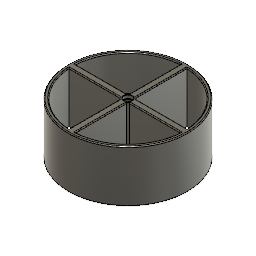
ExtrudedWheel v2 (Autodesk Fusion 360 design; units mm, degrees)
Autodesk Fusion 360 part; units mm, degrees
sketch "Sketch6" plane through (0, 0, 0) normal (0, 1, 0) x (1, 0, 0)
  circle A0 centre (0, 0) radius 73.5
  circle A1 centre (0, 0) radius 7
  circle A2 centre (0, 0) radius 71
  line L0 (4, 70.9044) -> (-4, 70.9044)
  line L1 (-4, 70.9044) -> (-4, -70.9044)
  line L2 (-4, -70.9044) -> (4, -70.9044)
  line L3 (4, -70.9044) -> (4, 70.9044)
  line L4 (4, 70.9044) -> (-4, -70.9044) construction
  line L5 (-4, 70.9044) -> (4, -70.9044) construction
  line L6 (72.9182, 4) -> (-72.9182, 4)
  line L7 (-72.9182, 4) -> (-72.9182, -4)
  line L8 (-72.9182, -4) -> (72.9182, -4)
  line L9 (72.9182, -4) -> (72.9182, 4)
  line L10 (72.9182, 4) -> (-72.9182, -4) construction
  line L11 (-72.9182, 4) -> (72.9182, -4) construction
  circle A3 centre (0, 0) radius 69
  dimension "d17" = 147
  dimension "d18" = 14
  dimension "d19" = 142
  dimension "d20" = 8
  dimension "d21" = 8
  dimension "d22" = 138
  measures "d17" diameter of A0
  measures "d18" diameter of A1
  measures "d19" diameter of A2
  measures "d22" diameter of A3
extrude "Extrude3" add sketch "Sketch6" along normal blind 64 contours A0 | A1 L3 L6 L8 | A1 L6 L8 A3 | A1 L3 L6 | A1 L3 L8 | A1 L1 L3 L6 | A1 L1 L3 A3 | A2 L3 L6 A3 | A2 L6 L8 A3 | L1 L3 L6 L8 | A1 L1 L3 A3 | A1 L1 L3 L8 | A2 L3 L8 A3 | A1 L1 L6 | A2 L0 L1 L3 A3 | A2 L6 L8 L9 | A1 L1 L6 L8 | A1 L1 L8 | A2 L1 L2 L3 A3 | A1 L6 L8 A3 | A2 L1 L6 A3 | A2 L0 L3 | A2 L1 L8 A3 | A2 L2 L3 | A2 L6 L8 A3 | A2 L0 L1 | A2 L0 | A2 L1 L2 | A2 L2 | A2 L6 L7 L8
hole "Hole2" at (0, 64, 0) direction (0, -1, 0) diameter 8.2 depth 64 tip angle 180
hole "Hole3" at (0, 64, 0) direction (0, -1, 0) diameter 10.2 depth 4 tip angle 180
fillet "Fillet1" radius 0.4 1 edges at (1.8442, 64, -4.7549)
fillet "Fillet2" radius 0.4 1 edges at (-1.4826, 60, -3.8225)
fillet "Fillet3" radius 1 8 edges at (-37.3143, 64, -4) (-37.3143, 64, 4) (-4, 64, 37.3143) (4, 64, 37.3143) (37.3143, 64, 4) (37.3143, 64, -4) (4, 64, -37.3143) (-4, 64, -37.3143)
fillet "Fillet4" radius 1 4 edges at (-48.7904, 64, 48.7904) (48.7904, 64, 48.7904) (48.7904, 0, -48.7904) (-48.7904, 64, -48.7904)
fillet "Fillet5" radius 1 1 edges at (48.7904, 64, -48.7904)
fillet "Fillet6" radius 1 1 edges at (-68.5261, 64, 26.5787)
fillet "Fillet7" radius 1 1 edges at (-68.5261, 0, 26.5787)
fillet "Fillet8" radius 1 8 edges at (37.3143, 0, 4) (4, 0, 37.3143) (-4, 0, 37.3143) (-37.3143, 0, 4) (-37.3143, 0, -4) (-4, 0, -37.3143) (4, 0, -37.8151) (37.8151, 0, -4)
fillet "Fillet9" radius 0.4 1 edges at (-1.4826, 0, -3.8225)
fillet "Fillet10" radius 1 3 edges at (-48.7904, 0, 48.7904) (-48.7904, 0, -48.7904) (48.7904, 0, 48.7904)
